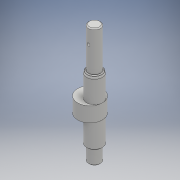
# Autodesk Inventor part: 3강
Saved by Autodesk Inventor 2018.3 (Build 223284000, 284)
## iProperties
Created: 2019-10-11
Part Number: 3강
Material: 일반
Document SubType Name: Modeling
Designer: MyTool
Density: 1 g/cm^3
Appearance: 기본값
Author: MyTool
Autodesk Inventor part; units mm, degrees
ref_plane "YZ Plane" through (0, 0, 0) normal (1, 0, 0) x (0, 1, 0)
ref_plane "XZ Plane" through (0, 0, 0) normal (0, 1, 0) x (-1, 0, 0)
ref_plane "XY Plane" through (0, 0, 0) normal (0, 0, 1) x (1, 0, 0)
sketch "스케치1" plane through (0, 0, 0) normal (1, 0, 0) x (0, 1, 0)
  line L0 (0, 0) -> (6, 0)
  line L1 (6, 0) -> (6, 15)
  line L2 (6, 15) -> (0, 15)
  line L3 (0, 15) -> (0, 0)
  line L4 (0, 15) -> (8, 15)
  line L5 (8, 15) -> (8, 40)
  line L6 (8, 40) -> (0, 40)
  line L7 (0, 40) -> (0, 15)
  line L8 (0, 40) -> (17, 40)
  line L9 (17, 40) -> (17, 55)
  line L10 (17, 55) -> (0, 55)
  line L11 (0, 55) -> (0, 40)
  line L12 (0, 55) -> (8, 55)
  line L13 (8, 55) -> (8, 80)
  line L14 (8, 80) -> (0, 80)
  line L15 (0, 80) -> (0, 55)
  line L16 (0, 80) -> (6, 80)
  line L17 (6, 80) -> (6, 120)
  line L18 (6, 120) -> (0, 120)
  line L19 (0, 120) -> (0, 80)
  dimension "d0" = 12
  dimension "d1" = 16
  dimension "d2" = 34
  dimension "d3" = 16
  dimension "d4" = 15
  dimension "d5" = 25
  dimension "d6" = 15
  dimension "d7" = 25
  dimension "d9" = 40
  dimension "d10" = 12
  constraints: 40 end point, 10 parallel, 5 horizontal, 5 perpendicular
  measures "d0" diameter of L1 L3
  measures "d1" diameter of L5 L7
  measures "d2" diameter of L9 L11
  measures "d3" diameter of L13 L15
  measures "d4" distance between parallel lines of L2 L0
  measures "d5" distance of L4.end L5.end
  measures "d6" distance between parallel lines of L10 L6
  measures "d7" distance between parallel lines of L14 L12
  measures "d9" distance between parallel lines of L14 L18
  measures "d10" diameter of L17 L19
revolve "회전1" add sketch "스케치1" angle 360 about axis through (0, 0, 40) along (0, 0, -1)
sketch "스케치2" plane through (0, 0, 55) normal (0, 0, 1) x (1, 0, 0)
  circle A0 centre (0, 0) radius 8 projected
  circle A1 centre (-4.5, 0) radius 12.5
  circle A2 centre (0, 0) radius 17 projected
  point P0 (0, 0)
  dimension "d11" = 25
  constraints: 1 centre point, 1 tangent
  measures "d11" diameter of A1
extrude "돌출1" cut sketch "스케치2" against normal up to next contours A2
sketch "스케치3" plane through (0, 0, 0) normal (0, 0, -1) x (-1, 0, 0)
  circle A0 centre (0, 0) radius 2
  dimension "d14" = 4
  constraints: 1 centre point, 1 coincident
  measures "d14" diameter of A0
hole "구멍1" at (0, 0, 0) direction (0, 0, 1) diameter 3.242 depth 11.8 tip angle 118 thread size "M4x0.7" class "6H" standard "ANSI Metric M Profile"
sketch "스케치4" plane through (0, 0, 0) normal (1, 0, 0) x (0, 1, 0)
  line L0 (8, 78.2679) -> (8, 80)
  line L1 (8, 80) -> (7, 80)
  line L2 (7, 80) -> (8, 78.2679)
  line L3 (8, 80) -> (8, 55) projected
  line L4 (-8, 80) -> (8, 80) projected
  line L5 (0, -24) -> (0, 144) projected
  point P0 (0, 0)
  dimension "d22" = 30
  dimension "d23" = 1
  constraints: 6 end point, 1 perpendicular, 1 vertical
  measures "d22" angle of L2 L0
  measures "d23" distance of L0.end L1.end
revolve "회전2" cut sketch "스케치4" angle 360 about axis through (0, 0, -10) along (0, 0, 1)
fillet "모깎기1" radius 4 1 edges at (0, -8, 78.2679)
fillet "모깎기2" radius 1 1 edges at (0, -7, 80)
sketch "스케치5" plane through (0, 0, 0) normal (1, 0, 0) x (0, 1, 0)
  circle A0 centre (8.6, 98) radius 8
  line L0 (6, 120) -> (6, 80) projected
  point P0 (0, 0)
  dimension "d27" = 16
  dimension "d29" = 5.4
  dimension "d30" = 18
  constraints: 1 centre point
  measures "d27" diameter of A0
  measures "d29" distance edge to line of A0 L0
  measures "d30" vertical distance of L0.end A0.centre
extrude "돌출2" cut sketch "스케치5" along normal mid plane 3
sketch "스케치6" plane through (0, 0, 0) normal (1, 0, 0) x (0, 1, 0)
  line L0 (-4.5, 105) -> (-6, 105)
  line L1 (-6, 105) -> (-6, 103.5)
  line L2 (-6, 103.5) -> (-4.5, 105)
  line L3 (-6, 120) -> (-6, 80) projected
  point P0 (0, 0)
  dimension "d33" = 1.5
  dimension "d34" = 45
  dimension "d35" = 25
  constraints: 6 end point, 1 collinear, 1 horizontal, 1 perpendicular
  measures "d33" distance of L0.end L1.end
  measures "d34" angle of L0 L2
  measures "d35" distance from line of L3.end L0
revolve "회전3" cut sketch "스케치6" angle 360 about axis through (0, -4.5, 105) along (0, -1, 0)
chamfer "모따기1" distance 1 angle 45 3 edges at (0, -6, 120) (0, -8, 15) (0, -6, 0)
